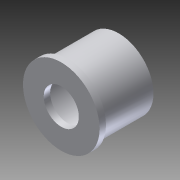
# Autodesk Inventor part: PVC Cap
Saved by Autodesk Inventor 2014 SP1 (Build 180222100, 222)
## iProperties
Created: 2012-02-19
Part Number: PVC Cap
Material: PVC-Piping
Document SubType Name: Modeling
Designer: Moses
Mass: 9.17625 g
Surface Area: 76.4542 cm^2
Volume: 6.55447 cm^3
Density: 1.4 g/cm^3
Appearance: Smooth - White
Author: Moses
Autodesk Inventor part; units mm, degrees
ref_plane "YZ Plane" through (0, 0, 0) normal (1, 0, 0) x (0, 1, 0)
ref_plane "XZ Plane" through (0, 0, 0) normal (0, 1, 0) x (-1, 0, 0)
ref_plane "XY Plane" through (0, 0, 0) normal (0, 0, 1) x (1, 0, 0)
sketch "Sketch1" plane through (0, 0, 0) normal (0, 0, 1) x (1, 0, 0)
  circle A0 centre (0, 0) radius 17.272
  circle A1 centre (0, 0) radius 19.05
  circle A2 centre (0, 0) radius 15.875
  dimension "d0" = 34.544
  dimension "d1" = 38.1
  dimension "d6" = 31.75
  constraints: 3 centre point, 3 coincident
  measures "d0" diameter of A0
  measures "d1" diameter of A1
  measures "d6" diameter of A2
extrude "Extrusion1" add sketch "Sketch1" along normal blind 3.175 contours A0 | A1 | A2
extrude "Extrusion2" add sketch "Sketch1" against normal blind 25.4 contours A0
sketch "Sketch2" plane through (0, 0, 3.175) normal (0, 0, 1) x (1, 0, 0)
  circle A0 centre (0, 0) radius 19.05 projected
  circle A1 centre (0, 0) radius 8.7313
  dimension "d7" = 17.4625
  constraints: 1 centre point, 1 coincident
  measures "d7" diameter of A1
extrude "Extrusion3" cut sketch "Sketch2" against normal blind 25.4 contours A1
body "Solid1"
